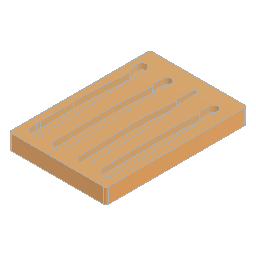
Tweezer-Carrier (Autodesk Fusion 360 design; units mm, degrees)
Autodesk Fusion 360 part; units mm, degrees
(part 1 of 2)
sketch "Sketch1" plane through (0, 0, 35.675) normal (0, 0, 1) x (-1, 0, 0)
  line L0 (-281.1, 293.942) -> (-205.1, 293.942)
  line L1 (-205.1, 293.942) -> (-205.1, 181.942)
  line L2 (-205.1, 181.942) -> (-281.1, 181.942)
  line L3 (-281.1, 181.942) -> (-281.1, 293.942)
  arc A0 (-205.1, 179.942) -> (-203.1, 181.942) centre (-205.1, 181.942) ccw
  line L4 (-203.1, 181.942) -> (-203.1, 293.942)
  arc A1 (-203.1, 293.942) -> (-205.1, 295.942) centre (-205.1, 293.942) ccw
  line L5 (-205.1, 295.942) -> (-281.1, 295.942)
  arc A2 (-281.1, 295.942) -> (-283.1, 293.942) centre (-281.1, 293.942) ccw
  line L6 (-283.1, 293.942) -> (-283.1, 181.942)
  arc A3 (-283.1, 181.942) -> (-281.1, 179.942) centre (-281.1, 181.942) ccw
  line L7 (-281.1, 179.942) -> (-205.1, 179.942)
  line L8 (-283.025, 293.942) -> (-283.025, 181.942)
  arc A4 (-283.025, 181.942) -> (-281.1, 180.017) centre (-281.1, 181.942) ccw
  line L9 (-281.1, 180.017) -> (-205.1, 180.017)
  arc A5 (-205.1, 180.017) -> (-203.175, 181.942) centre (-205.1, 181.942) ccw
  line L10 (-203.175, 181.942) -> (-203.175, 293.942)
  arc A6 (-203.175, 293.942) -> (-205.1, 295.867) centre (-205.1, 293.942) ccw
  line L11 (-205.1, 295.867) -> (-281.1, 295.867)
  arc A7 (-281.1, 295.867) -> (-283.025, 293.942) centre (-281.1, 293.942) ccw
  dimension "d162" = -0.075
extrude "Extrude1" add sketch "Sketch1" along normal blind 12.5 contours L0 L1 L2 L3 | L8 A4 L9 A5 L10 A6 L11 A7
sketch "Sketch2" plane through (0, 0, 48.175) normal (0, 0, 1) x (-1, 0, 0)
  arc A0 (-281.1, 295.867) -> (-283.025, 293.942) centre (-281.1, 293.942) ccw
  line L0 (-283.025, 293.942) -> (-283.025, 181.942)
  arc A1 (-283.025, 181.942) -> (-281.1, 180.017) centre (-281.1, 181.942) ccw
  line L1 (-281.1, 180.017) -> (-205.1, 180.017)
  arc A2 (-205.1, 180.017) -> (-203.175, 181.942) centre (-205.1, 181.942) ccw
  line L2 (-203.175, 181.942) -> (-203.175, 293.942)
  arc A3 (-203.175, 293.942) -> (-205.1, 295.867) centre (-205.1, 293.942) ccw
  line L3 (-205.1, 295.867) -> (-281.1, 295.867)
sketch "Sketch3" plane through (0, 0, 48.175) normal (0, 0, 1) x (-1, 0, 0)
  spline S0 degree 5 poles (-213.5459, 288.1293) (-213.4945, 288.1336) (-213.392, 288.1403) (-213.2392, 288.1448) (-213.0373, 288.1395) (-212.788, 288.1142) (-212.5418, 288.0705) (-212.2989, 288.0088) (-212.0595, 287.93) (-211.8239, 287.8356) (-211.5927, 287.7271) (-211.3661, 287.6064) (-211.1447, 287.475) (-210.929, 287.3345) (-210.7193, 287.1857) (-210.5161, 287.0295) (-210.3201, 286.8663) (-210.132, 286.6964) (-209.9529, 286.5201) (-209.7839, 286.3373) (-209.6265, 286.1478) (-209.4815, 285.9505) (-209.35, 285.7437) (-209.232, 285.5245) (-209.1273, 285.2896) (-209.0354, 285.0362) (-208.9554, 284.763) (-208.8863, 284.4709) (-208.8273, 284.1647) (-208.7775, 283.8515) (-208.7361, 283.5396) (-208.7023, 283.2363) (-208.6754, 282.9464) (-208.6547, 282.6709) (-208.6396, 282.4048) (-208.6295, 282.1406) (-208.6238, 281.8697) (-208.6217, 281.5848) (-208.6227, 281.2826) (-208.6261, 280.9654) (-208.6309, 280.64) (-208.6366, 280.3159) (-208.6424, 280.0035) (-208.6478, 279.713) (-208.6524, 279.4518) (-208.6559, 279.2244) (-208.6578, 279.0713) (-208.6586, 278.9729) (-208.6589, 278.9146) (-208.6591, 278.8873) knots 0 0 0 0 0 0 0.022222 0.044444 0.066667 0.088889 0.111111 0.133333 0.155556 0.177778 0.2 0.222222 0.244444 0.266667 0.288889 0.311111 0.333333 0.355556 0.377778 0.4 0.422222 0.444444 0.466667 0.488889 0.511111 0.533333 0.555556 0.577778 0.6 0.622222 0.644444 0.666667 0.688889 0.711111 0.733333 0.755556 0.777778 0.8 0.822222 0.844444 0.866667 0.888889 0.911111 0.933333 0.955556 0.977778 1 1 1 1 1 1
  spline S1 degree 5 poles (-208.6591, 278.8873) (-208.6588, 278.9046) (-208.6584, 278.9324) (-208.6579, 278.9537) (-208.6576, 278.9414) (-208.6579, 278.8572) (-208.6588, 278.7058) (-208.6603, 278.4928) (-208.6623, 278.2279) (-208.6648, 277.9222) (-208.6676, 277.5876) (-208.6708, 277.2352) (-208.6742, 276.8738) (-208.6778, 276.5093) (-208.6815, 276.1457) (-208.6854, 275.785) (-208.6886, 275.4997) (-208.691, 275.2877) (-208.6927, 275.1471) (-208.6935, 275.0771) knots 0 0 0 0 0 0 0.066667 0.133333 0.2 0.266667 0.333333 0.4 0.466667 0.533333 0.6 0.666667 0.733333 0.8 0.866667 0.933333 1 1 1 1 1 1
  spline S2 degree 5 poles (-208.6935, 275.0771) (-208.6936, 275.0186) (-208.6937, 274.9022) (-208.6943, 274.7292) (-208.6958, 274.5019) (-208.6987, 274.2215) (-208.7025, 273.9399) (-208.7066, 273.6464) (-208.7105, 273.3274) (-208.7137, 272.9745) (-208.7157, 272.59) (-208.717, 272.1953) (-208.7179, 271.82) (-208.7189, 271.4886) (-208.7196, 271.2097) (-208.719, 270.9594) (-208.7155, 270.6952) (-208.7074, 270.3748) (-208.6936, 269.977) (-208.6742, 269.5091) (-208.6496, 268.9944) (-208.6213, 268.4634) (-208.5907, 267.9451) (-208.56, 267.4558) (-208.5313, 266.9953) (-208.5068, 266.5529) (-208.488, 266.1123) (-208.4762, 265.6565) (-208.4715, 265.1727) (-208.4731, 264.6559) (-208.4796, 264.1063) (-208.489, 263.5285) (-208.4994, 262.9299) (-208.5091, 262.3195) (-208.5169, 261.7068) (-208.5219, 261.1003) (-208.5241, 260.5075) (-208.5234, 259.9343) (-208.5201, 259.3837) (-208.5145, 258.8563) (-208.507, 258.3486) (-208.4978, 257.8538) (-208.4873, 257.363) (-208.4756, 256.8669) (-208.463, 256.357) (-208.4498, 255.8268) (-208.4363, 255.2734) (-208.4229, 254.6965) (-208.4099, 254.0975) (-208.3977, 253.4794) (-208.3867, 252.8456) (-208.377, 252.1996) (-208.369, 251.5437) (-208.3628, 250.8798) (-208.3584, 250.2092) (-208.356, 249.5325) (-208.3555, 248.9866) (-208.3561, 248.5747) (-208.3569, 248.299) (-208.3573, 248.1609) knots 0 0 0 0 0 0 0.018182 0.036364 0.054545 0.072727 0.090909 0.109091 0.127273 0.145455 0.163636 0.181818 0.2 0.218182 0.236364 0.254545 0.272727 0.290909 0.309091 0.327273 0.345455 0.363636 0.381818 0.4 0.418182 0.436364 0.454545 0.472727 0.490909 0.509091 0.527273 0.545455 0.563636 0.581818 0.6 0.618182 0.636364 0.654545 0.672727 0.690909 0.709091 0.727273 0.745455 0.763636 0.781818 0.8 0.818182 0.836364 0.854545 0.872727 0.890909 0.909091 0.927273 0.945455 0.963636 0.981818 1 1 1 1 1 1
  spline S3 degree 5 poles (-208.3573, 248.1609) (-208.3602, 248.1208) (-208.3652, 248.0297) (-208.3703, 247.8598) (-208.3725, 247.5669) (-208.3678, 247.0952) (-208.3563, 246.533) (-208.3394, 245.9116) (-208.3191, 245.27) (-208.2977, 244.6446) (-208.2777, 244.0606) (-208.2614, 243.5208) (-208.251, 243.0003) (-208.2479, 242.4607) (-208.2534, 241.8621) (-208.2674, 241.1754) (-208.2891, 240.3959) (-208.3171, 239.54) (-208.3493, 238.6365) (-208.3839, 237.7205) (-208.4195, 236.8259) (-208.4555, 235.979) (-208.4923, 235.1896) (-208.532, 234.4502) (-208.5765, 233.7433) (-208.6279, 233.0464) (-208.6868, 232.339) (-208.7523, 231.6075) (-208.8209, 230.8526) (-208.8872, 230.0861) (-208.9456, 229.3261) (-208.991, 228.5915) (-209.0205, 227.8983) (-209.0343, 227.2537) (-209.0368, 226.6527) (-209.0348, 226.0821) (-209.0354, 225.5244) (-209.0449, 224.9611) (-209.0665, 224.3769) (-209.0999, 223.7617) (-209.143, 223.1093) (-209.1926, 222.4178) (-209.246, 221.6887) (-209.3016, 220.9271) (-209.3597, 220.1406) (-209.4214, 219.3378) (-209.488, 218.5274) (-209.5606, 217.7163) (-209.6393, 216.9087) (-209.7226, 216.1045) (-209.8074, 215.2995) (-209.8899, 214.4882) (-209.9662, 213.6659) (-210.033, 212.8304) (-210.0881, 211.9843) (-210.1314, 211.1375) (-210.1646, 210.3075) (-210.1912, 209.5148) (-210.2149, 208.7791) (-210.2394, 208.1151) (-210.2674, 207.5294) (-210.2999, 207.0151) (-210.3363, 206.5533) (-210.3747, 206.1204) (-210.4135, 205.6932) (-210.4514, 205.2566) (-210.4804, 204.8939) (-210.5014, 204.6132) (-210.515, 204.4223) (-210.5217, 204.3258) knots 0 0 0 0 0 0 0.01538462 0.03076923 0.04615385 0.06153846 0.07692308 0.09230769 0.10769231 0.12307692 0.13846154 0.15384615 0.16923077 0.18461538 0.2 0.21538462 0.23076923 0.24615385 0.26153846 0.27692308 0.29230769 0.30769231 0.32307692 0.33846154 0.35384615 0.36923077 0.38461538 0.4 0.41538462 0.43076923 0.44615385 0.46153846 0.47692308 0.49230769 0.50769231 0.52307692 0.53846154 0.55384615 0.56923077 0.58461538 0.6 0.61538462 0.63076923 0.64615385 0.66153846 0.67692308 0.69230769 0.70769231 0.72307692 0.73846154 0.75384615 0.76923077 0.78461538 0.8 0.81538462 0.83076923 0.84615385 0.86153846 0.87692308 0.89230769 0.90769231 0.92307692 0.93846154 0.95384615 0.96923077 0.98461538 1 1 1 1 1 1
  spline S4 degree 5 poles (-210.5217, 204.3258) (-210.5153, 204.3258) (-210.5025, 204.3257) (-210.4832, 204.3256) (-210.4576, 204.3254) (-210.4255, 204.3252) (-210.3998, 204.325) (-210.3805, 204.3248) (-210.3677, 204.3248) (-210.3613, 204.3247) knots 0 0 0 0 0 0 0.2 0.4 0.6 0.8 1 1 1 1 1 1
  spline S5 degree 5 poles (-233.3855, 288.3655) (-233.3109, 288.3868) (-233.1597, 288.4223) (-232.9269, 288.4544) (-232.6048, 288.4548) (-232.1838, 288.3864) (-231.7481, 288.2539) (-231.3053, 288.0677) (-230.8655, 287.8391) (-230.4388, 287.5764) (-230.0337, 287.2794) (-229.6557, 286.937) (-229.3093, 286.5403) (-229, 286.0916) (-228.7363, 285.6179) (-228.53, 285.1713) (-228.3889, 284.7958) (-228.3129, 284.5049) (-228.2864, 284.2462) (-228.2853, 283.9325) (-228.2909, 283.5017) (-228.2958, 282.9438) (-228.299, 282.279) (-228.3035, 281.5446) (-228.3126, 280.779) (-228.3271, 280.007) (-228.3456, 279.2426) (-228.3656, 278.4911) (-228.3842, 277.7515) (-228.3986, 277.0193) (-228.407, 276.2886) (-228.4091, 275.554) (-228.4051, 274.811) (-228.3963, 274.0567) (-228.384, 273.2907) (-228.3695, 272.5152) (-228.354, 271.7363) (-228.3381, 270.962) (-228.3224, 270.2004) (-228.307, 269.4576) (-228.2923, 268.7359) (-228.2782, 268.0318) (-228.2647, 267.3348) (-228.2518, 266.6317) (-228.2394, 265.9094) (-228.2275, 265.1587) (-228.2159, 264.3769) (-228.2046, 263.5719) (-228.1935, 262.7581) (-228.1826, 261.9529) (-228.1719, 261.1721) (-228.1613, 260.4259) (-228.1509, 259.715) (-228.1408, 259.0267) (-228.1311, 258.341) (-228.1219, 257.6352) (-228.1133, 256.8893) (-228.1054, 256.091) (-228.0982, 255.2416) (-228.0917, 254.3536) (-228.0858, 253.4464) (-228.0805, 252.542) (-228.0759, 251.6609) (-228.0719, 250.8182) (-228.0686, 250.019) (-228.0661, 249.2565) (-228.0646, 248.5169) (-228.0641, 247.7823) (-228.0646, 247.0346) (-228.066, 246.2591) (-228.0678, 245.4479) (-228.0694, 244.6008) (-228.0704, 243.723) (-228.07, 242.8238) (-228.0679, 241.9156) (-228.0637, 241.0121) (-228.0575, 240.1271) (-228.0496, 239.2735) (-228.0406, 238.461) (-228.0316, 237.6958) (-228.0235, 236.9786) (-228.0179, 236.3035) (-228.0161, 235.6561) (-228.0198, 235.0147) (-228.0301, 234.356) (-228.0478, 233.6596) (-228.0726, 232.913) (-228.1029, 232.1172) (-228.136, 231.2881) (-228.1687, 230.4489) (-228.1982, 229.6258) (-228.2224, 228.8413) (-228.2409, 228.1096) (-228.256, 227.4294) (-228.2719, 226.7838) (-228.2938, 226.1483) (-228.3263, 225.4969) (-228.3722, 224.8084) (-228.4309, 224.074) (-228.4985, 223.2987) (-228.5694, 222.4953) (-228.6375, 221.6812) (-228.6978, 220.8734) (-228.7474, 220.085) (-228.7877, 219.3194) (-228.823, 218.5722) (-228.8592, 217.8345) (-228.902, 217.0958) (-228.9558, 216.3473) (-229.0216, 215.5849) (-229.0961, 214.8119) (-229.1733, 214.0367) (-229.246, 213.2705) (-229.3073, 212.5252) (-229.3522, 211.8116) (-229.3792, 211.1364) (-229.3909, 210.5019) (-229.3919, 209.9061) (-229.3881, 209.3436) (-229.3851, 208.8058) (-229.387, 208.2812) (-229.3961, 207.7568) (-229.4141, 207.2199) (-229.4415, 206.6592) (-229.4788, 206.0671) (-229.5264, 205.439) (-229.5728, 204.906) (-229.6122, 204.4886) (-229.6406, 204.2026) (-229.6553, 204.0577) knots 0 0 0 0 0 0 0.008 0.016 0.024 0.032 0.04 0.048 0.056 0.064 0.072 0.08 0.088 0.096 0.104 0.112 0.12 0.128 0.136 0.144 0.152 0.16 0.168 0.176 0.184 0.192 0.2 0.208 0.216 0.224 0.232 0.24 0.248 0.256 0.264 0.272 0.28 0.288 0.296 0.304 0.312 0.32 0.328 0.336 0.344 0.352 0.36 0.368 0.376 0.384 0.392 0.4 0.408 0.416 0.424 0.432 0.44 0.448 0.456 0.464 0.472 0.48 0.488 0.496 0.504 0.512 0.52 0.528 0.536 0.544 0.552 0.56 0.568 0.576 0.584 0.592 0.6 0.608 0.616 0.624 0.632 0.64 0.648 0.656 0.664 0.672 0.68 0.688 0.696 0.704 0.712 0.72 0.728 0.736 0.744 0.752 0.76 0.768 0.776 0.784 0.792 0.8 0.808 0.816 0.824 0.832 0.84 0.848 0.856 0.864 0.872 0.88 0.888 0.896 0.904 0.912 0.92 0.928 0.936 0.944 0.952 0.96 0.968 0.976 0.984 0.992 1 1 1 1 1 1
  spline S6 degree 5 poles (-229.6553, 204.0577) (-229.6247, 204.0624) (-229.563, 204.0703) (-229.4689, 204.0774) (-229.3402, 204.0777) (-229.1753, 204.0615) (-229.0101, 204.0253) (-228.8525, 203.9625) (-228.7115, 203.8646) (-228.595, 203.723) (-228.5063, 203.5311) (-228.4442, 203.285) (-228.4052, 202.9837) (-228.3843, 202.6298) (-228.3765, 202.2298) (-228.3776, 201.7942) (-228.3842, 201.3354) (-228.3935, 200.8667) (-228.4033, 200.4009) (-228.412, 199.9484) (-228.4189, 199.5165) (-228.4236, 199.1069) (-228.4265, 198.7162) (-228.4282, 198.3371) (-228.4295, 197.9607) (-228.4311, 197.5782) (-228.4335, 197.1823) (-228.4368, 196.7698) (-228.4401, 196.3426) (-228.4429, 195.9069) (-228.4444, 195.4714) (-228.4451, 195.0458) (-228.4467, 194.6392) (-228.4527, 194.2582) (-228.4692, 193.9059) (-228.505, 193.58) (-228.5691, 193.2757) (-228.6686, 192.9873) (-228.8065, 192.7103) (-228.9798, 192.4437) (-229.1763, 192.1917) (-229.3792, 191.9626) (-229.5726, 191.7655) (-229.7468, 191.6078) (-229.9033, 191.493) (-230.0608, 191.4178) (-230.2434, 191.3746) (-230.4717, 191.3535) (-230.7492, 191.3447) (-231.0615, 191.3404) (-231.3856, 191.3348) (-231.6972, 191.3251) (-231.9778, 191.3124) (-232.2241, 191.3026) (-232.4476, 191.3053) (-232.6653, 191.3308) (-232.8945, 191.3882) (-233.144, 191.482) (-233.4112, 191.6116) (-233.6874, 191.7735) (-233.9599, 191.9626) (-234.2162, 192.1743) (-234.4471, 192.4064) (-234.6486, 192.6598) (-234.8203, 192.9367) (-234.9643, 193.24) (-235.0837, 193.572) (-235.1819, 193.9335) (-235.2611, 194.3223) (-235.3225, 194.7341) (-235.367, 195.1637) (-235.3953, 195.6055) (-235.4085, 196.0549) (-235.4082, 196.5085) (-235.3972, 196.9655) (-235.3794, 197.4284) (-235.3597, 197.9013) (-235.343, 198.3892) (-235.3344, 198.8963) (-235.3378, 199.4251) (-235.3563, 199.9749) (-235.3911, 200.5409) (-235.4414, 201.1126) (-235.5035, 201.673) (-235.5717, 202.2018) (-235.6389, 202.6781) (-235.6969, 203.0834) (-235.7369, 203.405) (-235.7502, 203.6386) (-235.7289, 203.7915) (-235.6658, 203.8856) (-235.5581, 203.9484) (-235.4111, 204.001) (-235.2393, 204.0517) (-235.0601, 204.1017) (-234.8882, 204.1493) (-234.7623, 204.1849) (-234.6755, 204.21) (-234.621, 204.2261) (-234.5946, 204.234) knots 0 0 0 0 0 0 0.01052632 0.02105263 0.03157895 0.04210526 0.05263158 0.06315789 0.07368421 0.08421053 0.09473684 0.10526316 0.11578947 0.12631579 0.13684211 0.14736842 0.15789474 0.16842105 0.17894737 0.18947368 0.2 0.21052632 0.22105263 0.23157895 0.24210526 0.25263158 0.26315789 0.27368421 0.28421053 0.29473684 0.30526316 0.31578947 0.32631579 0.33684211 0.34736842 0.35789474 0.36842105 0.37894737 0.38947368 0.4 0.41052632 0.42105263 0.43157895 0.44210526 0.45263158 0.46315789 0.47368421 0.48421053 0.49473684 0.50526316 0.51578947 0.52631579 0.53684211 0.54736842 0.55789474 0.56842105 0.57894737 0.58947368 0.6 0.61052632 0.62105263 0.63157895 0.64210526 0.65263158 0.66315789 0.67368421 0.68421053 0.69473684 0.70526316 0.71578947 0.72631579 0.73684211 0.74736842 0.75789474 0.76842105 0.77894737 0.78947368 0.8 0.81052632 0.82105263 0.83157895 0.84210526 0.85263158 0.86315789 0.87368421 0.88421053 0.89473684 0.90526316 0.91578947 0.92631579 0.93684211 0.94736842 0.95789474 0.96842105 0.97894737 0.98947368 1 1 1 1 1 1
  spline S7 degree 5 poles (-234.5946, 204.234) (-234.611, 204.3872) (-234.6431, 204.6936) (-234.6891, 205.1525) (-234.7462, 205.7631) (-234.8105, 206.525) (-234.8685, 207.2874) (-234.9212, 208.0541) (-234.9708, 208.8316) (-235.0201, 209.6287) (-235.0719, 210.4544) (-235.129, 211.3153) (-235.193, 212.2139) (-235.2642, 213.146) (-235.3411, 214.1003) (-235.4214, 215.0623) (-235.5025, 216.0167) (-235.5817, 216.9508) (-235.6574, 217.8567) (-235.7291, 218.7354) (-235.7979, 219.5944) (-235.8652, 220.445) (-235.933, 221.2984) (-236.0028, 222.1639) (-236.0759, 223.0445) (-236.1525, 223.9371) (-236.2325, 224.8356) (-236.3151, 225.733) (-236.3993, 226.6238) (-236.4834, 227.5063) (-236.566, 228.3848) (-236.6455, 229.2663) (-236.7204, 230.1594) (-236.79, 231.0718) (-236.8538, 232.008) (-236.9124, 232.9676) (-236.9672, 233.946) (-237.0195, 234.9362) (-237.0711, 235.9308) (-237.1234, 236.9227) (-237.1772, 237.9079) (-237.2328, 238.8861) (-237.2895, 239.8601) (-237.3464, 240.8345) (-237.4022, 241.815) (-237.4554, 242.8069) (-237.5043, 243.8142) (-237.5476, 244.8386) (-237.5838, 245.8798) (-237.6123, 246.9357) (-237.6326, 248.0024) (-237.645, 249.0741) (-237.6506, 250.144) (-237.6515, 251.2035) (-237.6503, 252.244) (-237.6499, 253.2578) (-237.6529, 254.2393) (-237.6618, 255.1862) (-237.6779, 256.1006) (-237.7014, 256.9906) (-237.7315, 257.8675) (-237.7666, 258.7431) (-237.8049, 259.6271) (-237.8443, 260.524) (-237.883, 261.4301) (-237.9195, 262.334) (-237.9529, 263.2222) (-237.9823, 264.0827) (-238.0071, 264.9091) (-238.0273, 265.7056) (-238.043, 266.4885) (-238.0547, 267.2803) (-238.0632, 268.1032) (-238.0699, 268.9747) (-238.0766, 269.9005) (-238.0854, 270.8726) (-238.0983, 271.8754) (-238.1168, 272.8894) (-238.1416, 273.8964) (-238.1718, 274.8836) (-238.2048, 275.849) (-238.2366, 276.8006) (-238.2628, 277.75) (-238.2798, 278.7077) (-238.2863, 279.6776) (-238.2836, 280.652) (-238.2775, 281.6054) (-238.2741, 282.5022) (-238.2746, 283.3085) (-238.2692, 284.003) (-238.2338, 284.5855) (-238.1206, 285.0929) (-237.8801, 285.5783) (-237.4904, 286.0822) (-236.9907, 286.5999) (-236.4884, 287.0711) (-236.0878, 287.4297) (-235.8432, 287.6352) (-235.6805, 287.7263) (-235.4402, 287.7959) (-235.0162, 287.9058) (-234.4897, 288.0497) (-233.9816, 288.1936) (-233.5926, 288.3056) (-233.3855, 288.3655) knots 0 0 0 0 0 0 0.01 0.02 0.03 0.04 0.05 0.06 0.07 0.08 0.09 0.1 0.11 0.12 0.13 0.14 0.15 0.16 0.17 0.18 0.19 0.2 0.21 0.22 0.23 0.24 0.25 0.26 0.27 0.28 0.29 0.3 0.31 0.32 0.33 0.34 0.35 0.36 0.37 0.38 0.39 0.4 0.41 0.42 0.43 0.44 0.45 0.46 0.47 0.48 0.49 0.5 0.51 0.52 0.53 0.54 0.55 0.56 0.57 0.58 0.59 0.6 0.61 0.62 0.63 0.64 0.65 0.66 0.67 0.68 0.69 0.7 0.71 0.72 0.73 0.74 0.75 0.76 0.77 0.78 0.79 0.8 0.81 0.82 0.83 0.84 0.85 0.86 0.87 0.88 0.89 0.9 0.91 0.92 0.93 0.94 0.95 0.96 0.97 0.98 0.99 1 1 1 1 1 1
  spline S8 degree 5 poles (-251.1217, 189.6278) (-251.0472, 189.6102) (-250.9024, 189.5836) (-250.6981, 189.57) (-250.4517, 189.6043) (-250.1865, 189.7344) (-249.9635, 189.951) (-249.7806, 190.2515) (-249.6345, 190.6314) (-249.5209, 191.0843) (-249.435, 191.6012) (-249.3718, 192.1712) (-249.3265, 192.7806) (-249.2947, 193.4137) (-249.2725, 194.0547) (-249.2564, 194.6891) (-249.2436, 195.3058) (-249.2316, 195.8979) (-249.2186, 196.4656) (-249.2036, 197.0168) (-249.1858, 197.5643) (-249.1649, 198.1228) (-249.141, 198.7054) (-249.114, 199.3204) (-249.0841, 199.9682) (-249.051, 200.6379) (-249.015, 201.3107) (-248.9769, 201.9639) (-248.9389, 202.5743) (-248.9049, 203.1218) (-248.8809, 203.5929) (-248.8758, 203.9853) (-248.9006, 204.307) (-248.9666, 204.5713) (-249.0837, 204.7924) (-249.2583, 204.9804) (-249.4464, 205.1083) (-249.6151, 205.1923) (-249.7397, 205.243) (-249.8051, 205.267) knots 0 0 0 0 0 0 0.028571 0.057143 0.085714 0.114286 0.142857 0.171429 0.2 0.228571 0.257143 0.285714 0.314286 0.342857 0.371429 0.4 0.428571 0.457143 0.485714 0.514286 0.542857 0.571429 0.6 0.628571 0.657143 0.685714 0.714286 0.742857 0.771429 0.8 0.828571 0.857143 0.885714 0.914286 0.942857 0.971429 1 1 1 1 1 1
  spline S9 degree 5 poles (-251.1217, 189.6278) (-251.1499, 189.624) (-251.2071, 189.6195) (-251.295, 189.6225) (-251.4163, 189.6458) (-251.5742, 189.707) (-251.7369, 189.7994) (-251.9013, 189.9211) (-252.0626, 190.0696) (-252.2157, 190.2423) (-252.3559, 190.4377) (-252.4799, 190.656) (-252.5867, 190.8998) (-252.6764, 191.1726) (-252.7508, 191.4781) (-252.8118, 191.8188) (-252.862, 192.1952) (-252.9036, 192.6042) (-252.9386, 193.0404) (-252.9687, 193.4965) (-252.9955, 193.9646) (-253.0203, 194.4369) (-253.0442, 194.9067) (-253.0682, 195.3696) (-253.0929, 195.8239) (-253.119, 196.2718) (-253.1468, 196.7179) (-253.1765, 197.1684) (-253.2083, 197.6294) (-253.2421, 198.1065) (-253.278, 198.6031) (-253.3156, 199.1196) (-253.3548, 199.6524) (-253.3952, 200.1922) (-253.4367, 200.7266) (-253.4791, 201.2414) (-253.5224, 201.722) (-253.5672, 202.1554) (-253.614, 202.5316) (-253.6642, 202.8456) (-253.7194, 203.0986) (-253.782, 203.3) (-253.8534, 203.4641) (-253.9325, 203.6077) (-254.0145, 203.7468) (-254.0887, 203.8942) (-254.1425, 204.0571) (-254.165, 204.236) (-254.1513, 204.4219) (-254.105, 204.5968) (-254.033, 204.7416) (-253.9429, 204.8421) (-253.8384, 204.8979) (-253.7194, 204.9195) (-253.5842, 204.921) (-253.4313, 204.9125) (-253.2944, 204.9014) (-253.1834, 204.8915) (-253.1056, 204.8842) (-253.0659, 204.8803) knots 0 0 0 0 0 0 0.018182 0.036364 0.054545 0.072727 0.090909 0.109091 0.127273 0.145455 0.163636 0.181818 0.2 0.218182 0.236364 0.254545 0.272727 0.290909 0.309091 0.327273 0.345455 0.363636 0.381818 0.4 0.418182 0.436364 0.454545 0.472727 0.490909 0.509091 0.527273 0.545455 0.563636 0.581818 0.6 0.618182 0.636364 0.654545 0.672727 0.690909 0.709091 0.727273 0.745455 0.763636 0.781818 0.8 0.818182 0.836364 0.854545 0.872727 0.890909 0.909091 0.927273 0.945455 0.963636 0.981818 1 1 1 1 1 1
  spline S10 degree 5 poles (-254.3567, 288.4328) (-254.2692, 288.4344) (-254.0999, 288.435) (-253.8631, 288.4277) (-253.5819, 288.4019) (-253.2812, 288.3428) (-253.0109, 288.2568) (-252.7308, 288.1439) (-252.4023, 288.0034) (-252.0152, 287.8327) (-251.6003, 287.6276) (-251.2011, 287.3857) (-250.8556, 287.1087) (-250.5679, 286.8064) (-250.3163, 286.494) (-250.0745, 286.1853) (-249.8331, 285.8875) (-249.6104, 285.597) (-249.4318, 285.3025) (-249.3133, 284.987) (-249.2479, 284.6307) (-249.2178, 284.2158) (-249.2038, 283.7313) (-249.1952, 283.1778) (-249.1867, 282.5639) (-249.1773, 281.9027) (-249.1679, 281.2092) (-249.1592, 280.4964) (-249.1508, 279.7731) (-249.1416, 279.0453) (-249.13, 278.3165) (-249.1148, 277.588) (-249.095, 276.8599) (-249.0707, 276.1315) (-249.0427, 275.4016) (-249.0128, 274.6687) (-248.9827, 273.9308) (-248.954, 273.186) (-248.9281, 272.432) (-248.9055, 271.6667) (-248.8861, 270.8883) (-248.8691, 270.0962) (-248.8536, 269.2911) (-248.8387, 268.4757) (-248.8235, 267.6557) (-248.8076, 266.8397) (-248.7911, 266.0396) (-248.7743, 265.2672) (-248.7576, 264.5324) (-248.7415, 263.841) (-248.7264, 263.1922) (-248.7124, 262.5757) (-248.6991, 261.9726) (-248.6859, 261.3621) (-248.6721, 260.727) (-248.6568, 260.0595) (-248.639, 259.368) (-248.6176, 258.6784) (-248.5921, 258.0229) (-248.5623, 257.4313) (-248.5288, 256.9218) (-248.4934, 256.4907) (-248.4588, 256.1082) (-248.428, 255.7346) (-248.4038, 255.333) (-248.3877, 254.8846) (-248.3801, 254.3856) (-248.3804, 253.8412) (-248.3866, 253.2609) (-248.396, 252.6524) (-248.405, 252.0222) (-248.4103, 251.375) (-248.4092, 250.7137) (-248.4001, 250.0399) (-248.3831, 249.3533) (-248.3598, 248.6526) (-248.3326, 247.9357) (-248.3042, 247.2005) (-248.2771, 246.4453) (-248.2529, 245.6693) (-248.2322, 244.873) (-248.2147, 244.0583) (-248.1998, 243.2279) (-248.1863, 242.386) (-248.1734, 241.5373) (-248.1602, 240.6875) (-248.1467, 239.8433) (-248.1333, 239.0113) (-248.1208, 238.1977) (-248.1102, 237.4074) (-248.1024, 236.6433) (-248.0985, 235.9055) (-248.0991, 235.1903) (-248.1046, 234.4905) (-248.115, 233.7969) (-248.1303, 233.0997) (-248.1503, 232.3903) (-248.1746, 231.6624) (-248.2029, 230.9141) (-248.2349, 230.1474) (-248.2706, 229.3665) (-248.3095, 228.5769) (-248.3516, 227.7842) (-248.3968, 226.9926) (-248.4448, 226.2039) (-248.4957, 225.417) (-248.5493, 224.6295) (-248.6053, 223.8383) (-248.6633, 223.0405) (-248.7227, 222.2346) (-248.7826, 221.4216) (-248.8418, 220.6052) (-248.8991, 219.7906) (-248.9532, 218.9837) (-249.0032, 218.1893) (-249.0486, 217.4108) (-249.0892, 216.6484) (-249.1261, 215.8979) (-249.1604, 215.1523) (-249.194, 214.4033) (-249.2286, 213.6431) (-249.2657, 212.8663) (-249.3063, 212.0713) (-249.351, 211.2625) (-249.3992, 210.4493) (-249.4502, 209.6443) (-249.503, 208.8616) (-249.5565, 208.1154) (-249.6095, 207.4182) (-249.6612, 206.779) (-249.7113, 206.2032) (-249.7498, 205.7953) (-249.7778, 205.5195) (-249.7961, 205.349) (-249.8051, 205.267) knots 0 0 0 0 0 0 0.00769231 0.01538462 0.02307692 0.03076923 0.03846154 0.04615385 0.05384615 0.06153846 0.06923077 0.07692308 0.08461538 0.09230769 0.1 0.10769231 0.11538462 0.12307692 0.13076923 0.13846154 0.14615385 0.15384615 0.16153846 0.16923077 0.17692308 0.18461538 0.19230769 0.2 0.20769231 0.21538462 0.22307692 0.23076923 0.23846154 0.24615385 0.25384615 0.26153846 0.26923077 0.27692308 0.28461538 0.29230769 0.3 0.30769231 0.31538462 0.32307692 0.33076923 0.33846154 0.34615385 0.35384615 0.36153846 0.36923077 0.37692308 0.38461538 0.39230769 0.4 0.40769231 0.41538462 0.42307692 0.43076923 0.43846154 0.44615385 0.45384615 0.46153846 0.46923077 0.47692308 0.48461538 0.49230769 0.5 0.50769231 0.51538462 0.52307692 0.53076923 0.53846154 0.54615385 0.55384615 0.56153846 0.56923077 0.57692308 0.58461538 0.59230769 0.6 0.60769231 0.61538462 0.62307692 0.63076923 0.63846154 0.64615385 0.65384615 0.66153846 0.66923077 0.67692308 0.68461538 0.69230769 0.7 0.70769231 0.71538462 0.72307692 0.73076923 0.73846154 0.74615385 0.75384615 0.76153846 0.76923077 0.77692308 0.78461538 0.79230769 0.8 0.80769231 0.81538462 0.82307692 0.83076923 0.83846154 0.84615385 0.85384615 0.86153846 0.86923077 0.87692308 0.88461538 0.89230769 0.9 0.90769231 0.91538462 0.92307692 0.93076923 0.93846154 0.94615385 0.95384615 0.96153846 0.96923077 0.97692308 0.98461538 0.99230769 1 1 1 1 1 1
  spline S11 degree 5 poles (-254.3567, 288.4328) (-254.4631, 288.4521) (-254.6744, 288.4769) (-254.9863, 288.4731) (-255.3923, 288.3858) (-255.8836, 288.1455) (-256.3585, 287.7914) (-256.8175, 287.3595) (-257.2594, 286.8952) (-257.6798, 286.4374) (-258.0685, 286.0052) (-258.4081, 285.5834) (-258.6806, 285.1414) (-258.8736, 284.6485) (-258.9884, 284.0953) (-259.0387, 283.4922) (-259.0431, 282.8563) (-259.0202, 282.2018) (-258.9823, 281.5295) (-258.9378, 280.8333) (-258.8912, 280.1052) (-258.845, 279.3403) (-258.8008, 278.5431) (-258.7592, 277.7238) (-258.7203, 276.8948) (-258.6838, 276.0664) (-258.6495, 275.243) (-258.617, 274.4197) (-258.586, 273.5857) (-258.5562, 272.7284) (-258.5273, 271.8367) (-258.4986, 270.905) (-258.4696, 269.9362) (-258.4394, 268.94) (-258.4072, 267.9291) (-258.3727, 266.917) (-258.3353, 265.9147) (-258.2953, 264.9282) (-258.2532, 263.9562) (-258.2099, 262.9923) (-258.1663, 262.0276) (-258.1232, 261.0529) (-258.0812, 260.0612) (-258.0401, 259.0498) (-257.9995, 258.0219) (-257.9584, 256.9845) (-257.9159, 255.9467) (-257.8711, 254.9181) (-257.8237, 253.9075) (-257.774, 252.9208) (-257.7233, 251.9603) (-257.6732, 251.0251) (-257.6253, 250.1119) (-257.5814, 249.2159) (-257.5424, 248.3309) (-257.5086, 247.4502) (-257.4794, 246.5673) (-257.4537, 245.6766) (-257.43, 244.774) (-257.4067, 243.8578) (-257.3825, 242.9293) (-257.356, 241.993) (-257.3264, 241.0557) (-257.2928, 240.125) (-257.2545, 239.2086) (-257.2109, 238.313) (-257.1612, 237.4426) (-257.1048, 236.5992) (-257.0412, 235.7818) (-256.9698, 234.9862) (-256.8903, 234.2049) (-256.8026, 233.4266) (-256.7069, 232.638) (-256.6035, 231.8264) (-256.4935, 230.9824) (-256.3782, 230.1018) (-256.2596, 229.1887) (-256.14, 228.253) (-256.0215, 227.3069) (-255.9059, 226.3626) (-255.7941, 225.429) (-255.6856, 224.5091) (-255.5788, 223.5984) (-255.4713, 222.6885) (-255.3607, 221.7693) (-255.2445, 220.8318) (-255.1213, 219.8707) (-254.991, 218.8868) (-254.8544, 217.8861) (-254.7132, 216.8776) (-254.5695, 215.8717) (-254.4255, 214.8779) (-254.2831, 213.9034) (-254.1435, 212.951) (-254.0076, 212.0199) (-253.8757, 211.1067) (-253.7479, 210.2069) (-253.6243, 209.3153) (-253.5046, 208.428) (-253.3889, 207.5421) (-253.277, 206.656) (-253.1906, 205.9464) (-253.1276, 205.4136) (-253.0863, 205.0581) (-253.0659, 204.8803) knots 0 0 0 0 0 0 0.01 0.02 0.03 0.04 0.05 0.06 0.07 0.08 0.09 0.1 0.11 0.12 0.13 0.14 0.15 0.16 0.17 0.18 0.19 0.2 0.21 0.22 0.23 0.24 0.25 0.26 0.27 0.28 0.29 0.3 0.31 0.32 0.33 0.34 0.35 0.36 0.37 0.38 0.39 0.4 0.41 0.42 0.43 0.44 0.45 0.46 0.47 0.48 0.49 0.5 0.51 0.52 0.53 0.54 0.55 0.56 0.57 0.58 0.59 0.6 0.61 0.62 0.63 0.64 0.65 0.66 0.67 0.68 0.69 0.7 0.71 0.72 0.73 0.74 0.75 0.76 0.77 0.78 0.79 0.8 0.81 0.82 0.83 0.84 0.85 0.86 0.87 0.88 0.89 0.9 0.91 0.92 0.93 0.94 0.95 0.96 0.97 0.98 0.99 1 1 1 1 1 1
  spline S12 degree 5 poles (-272.7173, 288.4864) (-272.632, 288.5001) (-272.46, 288.5217) (-272.1981, 288.5368) (-271.8414, 288.5221) (-271.3844, 288.4468) (-270.9205, 288.3177) (-270.4587, 288.1409) (-270.0122, 287.9255) (-269.5941, 287.6792) (-269.2145, 287.4068) (-268.8764, 287.1055) (-268.5772, 286.7677) (-268.3121, 286.3852) (-268.0771, 285.9539) (-267.8719, 285.4771) (-267.6981, 284.9625) (-267.557, 284.4199) (-267.449, 283.8585) (-267.3712, 283.2847) (-267.3187, 282.7026) (-267.2859, 282.1141) (-267.2672, 281.5201) (-267.2578, 280.9201) (-267.2546, 280.3131) (-267.2552, 279.6981) (-267.2579, 279.0741) (-267.2614, 278.4406) (-267.2644, 277.7981) (-267.2659, 277.1479) (-267.265, 276.4918) (-267.2612, 275.8315) (-267.2541, 275.1689) (-267.244, 274.5056) (-267.2315, 273.8426) (-267.2173, 273.1803) (-267.2022, 272.5187) (-267.187, 271.8569) (-267.1722, 271.1931) (-267.1582, 270.5251) (-267.1453, 269.8513) (-267.1335, 269.1706) (-267.1225, 268.4839) (-267.112, 267.7939) (-267.1016, 267.1054) (-267.0906, 266.4231) (-267.0786, 265.7513) (-267.0654, 265.0924) (-267.0509, 264.4458) (-267.0356, 263.8079) (-267.0201, 263.1741) (-267.0053, 262.5394) (-266.9924, 261.9003) (-266.9829, 261.256) (-266.9783, 260.6084) (-266.9797, 259.96) (-266.9874, 259.3133) (-267.0006, 258.669) (-267.0169, 258.0252) (-267.0328, 257.377) (-267.0445, 256.7196) (-267.0489, 256.0487) (-267.0444, 255.3626) (-267.0316, 254.6641) (-267.0134, 253.9593) (-266.9935, 253.2561) (-266.9756, 252.5618) (-266.9625, 251.8818) (-266.9551, 251.2173) (-266.9516, 250.5648) (-266.9493, 249.9177) (-266.9452, 249.2679) (-266.937, 248.6073) (-266.9241, 247.9291) (-266.9082, 247.2294) (-266.8921, 246.5071) (-266.8789, 245.7652) (-266.8715, 245.0106) (-266.8715, 244.2552) (-266.8782, 243.5163) (-266.8895, 242.8129) (-266.9029, 242.1609) (-266.9156, 241.5689) (-266.926, 241.0339) (-266.9339, 240.5355) (-266.941, 240.0414) (-266.9494, 239.5174) (-266.9612, 238.9348) (-266.9777, 238.2816) (-266.9992, 237.5612) (-267.0256, 236.7877) (-267.0561, 235.981) (-267.0897, 235.1628) (-267.1251, 234.3519) (-267.1612, 233.56) (-267.1971, 232.7932) (-267.2318, 232.0528) (-267.2644, 231.3361) (-267.2943, 230.6376) (-267.3211, 229.9495) (-267.3444, 229.2631) (-267.3641, 228.5694) (-267.3805, 227.8602) (-267.3939, 227.1286) (-267.405, 226.3705) (-267.4148, 225.5849) (-267.4244, 224.7737) (-267.4353, 223.9407) (-267.4485, 223.0913) (-267.4652, 222.2311) (-267.4863, 221.3663) (-267.5122, 220.5018) (-267.5432, 219.642) (-267.5791, 218.7898) (-267.6196, 217.9472) (-267.6642, 217.1148) (-267.7122, 216.2918) (-267.7629, 215.4757) (-267.8155, 214.6629) (-267.8693, 213.849) (-267.9234, 213.0304) (-267.9772, 212.2051) (-268.0301, 211.3734) (-268.0816, 210.5391) (-268.1316, 209.7103) (-268.1797, 208.8975) (-268.2261, 208.1133) (-268.2708, 207.3698) (-268.3137, 206.6784) (-268.3549, 206.0479) (-268.3946, 205.4834) (-268.425, 205.0866) (-268.4471, 204.8203) (-268.4616, 204.6566) (-268.4687, 204.5782) knots 0 0 0 0 0 0 0.00769231 0.01538462 0.02307692 0.03076923 0.03846154 0.04615385 0.05384615 0.06153846 0.06923077 0.07692308 0.08461538 0.09230769 0.1 0.10769231 0.11538462 0.12307692 0.13076923 0.13846154 0.14615385 0.15384615 0.16153846 0.16923077 0.17692308 0.18461538 0.19230769 0.2 0.20769231 0.21538462 0.22307692 0.23076923 0.23846154 0.24615385 0.25384615 0.26153846 0.26923077 0.27692308 0.28461538 0.29230769 0.3 0.30769231 0.31538462 0.32307692 0.33076923 0.33846154 0.34615385 0.35384615 0.36153846 0.36923077 0.37692308 0.38461538 0.39230769 0.4 0.40769231 0.41538462 0.42307692 0.43076923 0.43846154 0.44615385 0.45384615 0.46153846 0.46923077 0.47692308 0.48461538 0.49230769 0.5 0.50769231 0.51538462 0.52307692 0.53076923 0.53846154 0.54615385 0.55384615 0.56153846 0.56923077 0.57692308 0.58461538 0.59230769 0.6 0.60769231 0.61538462 0.62307692 0.63076923 0.63846154 0.64615385 0.65384615 0.66153846 0.66923077 0.67692308 0.68461538 0.69230769 0.7 0.70769231 0.71538462 0.72307692 0.73076923 0.73846154 0.74615385 0.75384615 0.76153846 0.76923077 0.77692308 0.78461538 0.79230769 0.8 0.80769231 0.81538462 0.82307692 0.83076923 0.83846154 0.84615385 0.85384615 0.86153846 0.86923077 0.87692308 0.88461538 0.89230769 0.9 0.90769231 0.91538462 0.92307692 0.93076923 0.93846154 0.94615385 0.95384615 0.96153846 0.96923077 0.97692308 0.98461538 0.99230769 1 1 1 1 1 1
  spline S13 degree 5 poles (-272.7173, 288.4864) (-272.8609, 288.4558) (-273.1449, 288.3876) (-273.5613, 288.2648) (-274.0971, 288.06) (-274.7313, 287.7342) (-275.3194, 287.3346) (-275.8397, 286.8531) (-276.2682, 286.2793) (-276.5882, 285.6026) (-276.8025, 284.8146) (-276.9294, 283.9115) (-276.9938, 282.8973) (-277.0205, 281.7862) (-277.0261, 280.6059) (-277.0209, 279.3903) (-277.0101, 278.173) (-276.9953, 276.9802) (-276.9764, 275.8237) (-276.9527, 274.6943) (-276.9233, 273.5703) (-276.8876, 272.4251) (-276.8459, 271.2354) (-276.7998, 269.9896) (-276.752, 268.6934) (-276.7062, 267.3637) (-276.6661, 266.023) (-276.6346, 264.6938) (-276.6131, 263.3929) (-276.6009, 262.1257) (-276.5953, 260.8864) (-276.5928, 259.6636) (-276.5895, 258.4428) (-276.5818, 257.2108) (-276.5678, 255.9598) (-276.5467, 254.6881) (-276.5191, 253.3978) (-276.4861, 252.0927) (-276.4487, 250.7759) (-276.408, 249.448) (-276.3642, 248.1051) (-276.3174, 246.7412) (-276.2672, 245.3503) (-276.2136, 243.9288) (-276.1564, 242.4774) (-276.0965, 241.0039) (-276.0348, 239.5236) (-275.9729, 238.0552) (-275.9117, 236.6174) (-275.8517, 235.2254) (-275.7925, 233.8875) (-275.7322, 232.6009) (-275.6674, 231.3506) (-275.5943, 230.115) (-275.5092, 228.8705) (-275.4097, 227.5962) (-275.2951, 226.2788) (-275.1678, 224.9172) (-275.0317, 223.5195) (-274.892, 222.0997) (-274.7538, 220.674) (-274.6217, 219.258) (-274.4985, 217.863) (-274.3845, 216.4933) (-274.2787, 215.1483) (-274.1786, 213.8238) (-274.0812, 212.5135) (-273.9836, 211.2107) (-273.8835, 209.9103) (-273.7793, 208.6086) (-273.6701, 207.3036) (-273.5784, 206.2562) (-273.5071, 205.4686) (-273.4585, 204.9425) (-273.4339, 204.6793) knots 0 0 0 0 0 0 0.01428571 0.02857143 0.04285714 0.05714286 0.07142857 0.08571429 0.1 0.11428571 0.12857143 0.14285714 0.15714286 0.17142857 0.18571429 0.2 0.21428571 0.22857143 0.24285714 0.25714286 0.27142857 0.28571429 0.3 0.31428571 0.32857143 0.34285714 0.35714286 0.37142857 0.38571429 0.4 0.41428571 0.42857143 0.44285714 0.45714286 0.47142857 0.48571429 0.5 0.51428571 0.52857143 0.54285714 0.55714286 0.57142857 0.58571429 0.6 0.61428571 0.62857143 0.64285714 0.65714286 0.67142857 0.68571429 0.7 0.71428571 0.72857143 0.74285714 0.75714286 0.77142857 0.78571429 0.8 0.81428571 0.82857143 0.84285714 0.85714286 0.87142857 0.88571429 0.9 0.91428571 0.92857143 0.94285714 0.95714286 0.97142857 0.98571429 1 1 1 1 1 1
  spline S14 degree 5 poles (-268.4687, 204.5782) (-268.435, 204.571) (-268.3676, 204.5553) (-268.2667, 204.5282) (-268.1326, 204.4852) (-267.9668, 204.4186) (-267.8066, 204.3358) (-267.6596, 204.23) (-267.5337, 204.0936) (-267.4347, 203.9206) (-267.3631, 203.7088) (-267.3162, 203.4582) (-267.2893, 203.1698) (-267.2776, 202.8436) (-267.2774, 202.4783) (-267.2853, 202.0724) (-267.2986, 201.6247) (-267.3147, 201.136) (-267.3316, 200.6089) (-267.3469, 200.0498) (-267.3587, 199.4678) (-267.3657, 198.8736) (-267.3672, 198.2788) (-267.3635, 197.6947) (-267.3563, 197.1312) (-267.349, 196.5959) (-267.3466, 196.0933) (-267.3563, 195.6233) (-267.3864, 195.1828) (-267.4453, 194.7667) (-267.5401, 194.3698) (-267.6758, 193.9877) (-267.854, 193.618) (-268.072, 193.2622) (-268.3234, 192.925) (-268.6002, 192.6125) (-268.894, 192.3318) (-269.1976, 192.0896) (-269.5068, 191.8912) (-269.8213, 191.7393) (-270.1431, 191.6351) (-270.4752, 191.5785) (-270.8197, 191.5686) (-271.1765, 191.6049) (-271.5418, 191.6868) (-271.9096, 191.8139) (-272.2719, 191.9846) (-272.6205, 192.1962) (-272.9468, 192.4439) (-273.2439, 192.7206) (-273.506, 193.0173) (-273.7289, 193.3261) (-273.9106, 193.641) (-274.0507, 193.9597) (-274.1514, 194.2862) (-274.2171, 194.6301) (-274.2535, 195.0041) (-274.2673, 195.4208) (-274.2654, 195.8904) (-274.2543, 196.4177) (-274.2396, 196.9994) (-274.2255, 197.6254) (-274.2156, 198.2809) (-274.2125, 198.9483) (-274.2178, 199.609) (-274.2327, 200.2455) (-274.2576, 200.8435) (-274.2924, 201.393) (-274.3364, 201.8915) (-274.3885, 202.3431) (-274.4464, 202.7549) (-274.5063, 203.1337) (-274.5622, 203.4831) (-274.6059, 203.8003) (-274.6258, 204.0714) (-274.6092, 204.2763) (-274.5461, 204.401) (-274.4337, 204.4496) (-274.2799, 204.4539) (-274.0965, 204.4547) (-273.8926, 204.4827) (-273.7165, 204.5382) (-273.5778, 204.6006) (-273.4824, 204.6515) (-273.4339, 204.6793) knots 0 0 0 0 0 0 0.0125 0.025 0.0375 0.05 0.0625 0.075 0.0875 0.1 0.1125 0.125 0.1375 0.15 0.1625 0.175 0.1875 0.2 0.2125 0.225 0.2375 0.25 0.2625 0.275 0.2875 0.3 0.3125 0.325 0.3375 0.35 0.3625 0.375 0.3875 0.4 0.4125 0.425 0.4375 0.45 0.4625 0.475 0.4875 0.5 0.5125 0.525 0.5375 0.55 0.5625 0.575 0.5875 0.6 0.6125 0.625 0.6375 0.65 0.6625 0.675 0.6875 0.7 0.7125 0.725 0.7375 0.75 0.7625 0.775 0.7875 0.8 0.8125 0.825 0.8375 0.85 0.8625 0.875 0.8875 0.9 0.9125 0.925 0.9375 0.95 0.9625 0.975 0.9875 1 1 1 1 1 1
  spline S15 degree 5 poles (-215.0905, 203.3708) (-215.1465, 203.3929) (-215.2541, 203.4268) (-215.4024, 203.4475) (-215.5735, 203.4144) (-215.7432, 203.2715) (-215.8689, 203.0277) (-215.952, 202.6852) (-215.9948, 202.2483) (-216.0007, 201.7229) (-215.9747, 201.117) (-215.9235, 200.4405) (-215.8541, 199.7052) (-215.7737, 198.924) (-215.6881, 198.1112) (-215.6013, 197.2814) (-215.5139, 196.45) (-215.423, 195.6322) (-215.3209, 194.8435) (-215.1977, 194.0983) (-215.0418, 193.4102) (-214.8414, 192.7912) (-214.5856, 192.2513) (-214.2657, 191.7977) (-213.8767, 191.4346) (-213.4159, 191.1638) (-212.9892, 191.0213) (-212.6366, 190.9559) (-212.387, 190.9308) (-212.2586, 190.9228) knots 0 0 0 0 0 0 0.04 0.08 0.12 0.16 0.2 0.24 0.28 0.32 0.36 0.4 0.44 0.48 0.52 0.56 0.6 0.64 0.68 0.72 0.76 0.8 0.84 0.88 0.92 0.96 1 1 1 1 1 1
  spline S16 degree 5 poles (-210.3613, 204.3247) (-210.3119, 204.3026) (-210.2157, 204.255) (-210.0795, 204.1737) (-209.9138, 204.0454) (-209.733, 203.8512) (-209.5778, 203.621) (-209.4459, 203.3507) (-209.3343, 203.0346) (-209.2389, 202.6678) (-209.1549, 202.2476) (-209.0768, 201.7759) (-208.9993, 201.2587) (-208.9171, 200.7049) (-208.826, 200.1247) (-208.7229, 199.5283) (-208.6066, 198.9245) (-208.4784, 198.3192) (-208.3417, 197.716) (-208.2024, 197.1168) (-208.0684, 196.5226) (-207.9497, 195.9346) (-207.8583, 195.3546) (-207.8083, 194.7863) (-207.8147, 194.2351) (-207.8915, 193.7074) (-208.0488, 193.2105) (-208.291, 192.7513) (-208.6145, 192.3359) (-209.0048, 191.9691) (-209.4397, 191.6543) (-209.8942, 191.3933) (-210.3445, 191.1868) (-210.7726, 191.034) (-211.1712, 190.9331) (-211.545, 190.8811) (-211.8321, 190.8762) (-212.0455, 190.892) (-212.1876, 190.9111) (-212.2586, 190.9228) knots 0 0 0 0 0 0 0.028571 0.057143 0.085714 0.114286 0.142857 0.171429 0.2 0.228571 0.257143 0.285714 0.314286 0.342857 0.371429 0.4 0.428571 0.457143 0.485714 0.514286 0.542857 0.571429 0.6 0.628571 0.657143 0.685714 0.714286 0.742857 0.771429 0.8 0.828571 0.857143 0.885714 0.914286 0.942857 0.971429 1 1 1 1 1 1
  line L0 (-210.9023, 190.6998) -> (-213.6149, 191.1458)
  spline S17 degree 5 poles (-215.0905, 203.3708) (-215.0967, 203.4305) (-215.1086, 203.544) (-215.125, 203.697) (-215.1481, 203.9278) (-215.1925, 204.4704) (-215.257, 205.3143) (-215.34, 206.4055) (-215.436, 207.6291) (-215.538, 208.8568) (-215.6398, 209.993) (-215.7384, 211.017) (-215.8332, 211.9579) (-215.9251, 212.8749) (-216.0158, 213.8351) (-216.1073, 214.8932) (-216.2009, 216.0674) (-216.2971, 217.3438) (-216.3961, 218.6877) (-216.4974, 220.0525) (-216.6005, 221.3899) (-216.7042, 222.6587) (-216.8074, 223.836) (-216.9089, 224.9233) (-217.0076, 225.9378) (-217.1022, 226.9074) (-217.192, 227.863) (-217.2764, 228.833) (-217.3552, 229.8354) (-217.4287, 230.8787) (-217.4971, 231.964) (-217.5609, 233.0873) (-217.6203, 234.2416) (-217.6754, 235.4192) (-217.7257, 236.6134) (-217.7708, 237.8182) (-217.8102, 239.028) (-217.844, 240.2377) (-217.8725, 241.442) (-217.8968, 242.6358) (-217.919, 243.8135) (-217.9418, 244.9702) (-217.9676, 246.1022) (-217.9985, 247.208) (-218.0358, 248.2888) (-218.0792, 249.3497) (-218.1266, 250.4005) (-218.1747, 251.4531) (-218.22, 252.521) (-218.2589, 253.6165) (-218.2889, 254.7496) (-218.309, 255.9257) (-218.3203, 257.1454) (-218.3246, 258.4049) (-218.3247, 259.6967) (-218.3231, 261.0103) (-218.3221, 262.3327) (-218.3225, 263.6491) (-218.324, 264.9434) (-218.3248, 266.2004) (-218.3233, 267.4084) (-218.3179, 268.5612) (-218.3084, 269.6608) (-218.2963, 270.7193) (-218.286, 271.7623) (-218.2834, 272.8238) (-218.295, 273.9375) (-218.3257, 275.1286) (-218.378, 276.4052) (-218.4499, 277.7516) (-218.5336, 279.1166) (-218.6164, 280.4269) (-218.6832, 281.6055) (-218.7176, 282.5894) (-218.7046, 283.3472) (-218.6318, 283.8963) (-218.492, 284.3236) (-218.2828, 284.7402) (-218.0071, 285.2254) (-217.6728, 285.78) (-217.2893, 286.3617) (-216.8655, 286.9106) (-216.406, 287.3843) (-215.9112, 287.7606) (-215.38, 288.029) (-214.8106, 288.1858) (-214.3242, 288.2204) (-213.9419, 288.1948) (-213.6792, 288.1549) (-213.5459, 288.1293) knots 0 0 0 0 0 0 0.01176471 0.02352941 0.03529412 0.04705882 0.05882353 0.07058824 0.08235294 0.09411765 0.10588235 0.11764706 0.12941176 0.14117647 0.15294118 0.16470588 0.17647059 0.18823529 0.2 0.21176471 0.22352941 0.23529412 0.24705882 0.25882353 0.27058824 0.28235294 0.29411765 0.30588235 0.31764706 0.32941176 0.34117647 0.35294118 0.36470588 0.37647059 0.38823529 0.4 0.41176471 0.42352941 0.43529412 0.44705882 0.45882353 0.47058824 0.48235294 0.49411765 0.50588235 0.51764706 0.52941176 0.54117647 0.55294118 0.56470588 0.57647059 0.58823529 0.6 0.61176471 0.62352941 0.63529412 0.64705882 0.65882353 0.67058824 0.68235294 0.69411765 0.70588235 0.71764706 0.72941176 0.74117647 0.75294118 0.76470588 0.77647059 0.78823529 0.8 0.81176471 0.82352941 0.83529412 0.84705882 0.85882353 0.87058824 0.88235294 0.89411765 0.90588235 0.91764706 0.92941176 0.94117647 0.95294118 0.96470588 0.97647059 0.98823529 1 1 1 1 1 1
  line L1 (-214.2131, 194.906) -> (-215.9679, 211.8357)
  line L2 (-272.7009, 290.8399) -> (-212.8441, 290.422)
  line L3 (-272.7009, 290.8399) -> (-272.7173, 288.4864)
  line L4 (-254.3875, 290.7121) -> (-254.3567, 288.4328)
  line L5 (-232.7833, 288.3613) -> (-232.7679, 290.5611)
  point P0 (-212.3453, 288.0175)
  point P1 (-211.2196, 287.5177)
  point P2 (-210.2186, 286.7728)
  point P3 (-209.4421, 285.8841)
  point P4 (-208.9363, 284.6731)
  point P5 (-208.6797, 282.983)
  point P6 (-208.6225, 281.5739)
  point P7 (-208.646, 279.8075)
  point P8 (-208.6583, 278.8029)
  point P9 (-208.6698, 277.3427)
  point P10 (-208.7003, 274.1033)
  point P11 (-208.7137, 272.9195)
  point P12 (-208.719, 271.4346)
  point P13 (-208.7101, 270.4996)
  point P14 (-208.6018, 268.1386)
  point P15 (-208.4813, 265.8135)
  point P16 (-208.5032, 262.6805)
  point P17 (-208.5168, 259.1031)
  point P18 (-208.4639, 256.3956)
  point P19 (-208.3864, 252.8062)
  point P20 (-208.3653, 247.0227)
  point P21 (-208.2825, 244.192)
  point P22 (-208.2575, 241.7145)
  point P23 (-208.4397, 236.3586)
  point P24 (-208.7016, 232.1807)
  point P25 (-209.0136, 228.0004)
  point P26 (-209.0415, 225.241)
  point P27 (-209.2161, 222.0986)
  point P28 (-209.5958, 217.3629)
  point P29 (-210.068, 212.2684)
  point P30 (-210.2529, 207.8525)
  point P31 (-210.3881, 205.9735)
  point P32 (-209.67, 203.7483)
  point P33 (-209.2025, 202.4734)
  point P34 (-208.6977, 199.4079)
  point P35 (-207.9024, 195.6067)
  point P36 (-208.3694, 192.6755)
  point P37 (-210.6141, 191.0963)
  point P38 (-215.1484, 203.9503)
  point P39 (-215.5296, 208.7374)
  point P40 (-216.0346, 214.0676)
  point P41 (-216.6786, 222.3332)
  point P42 (-217.2124, 228.1101)
  point P43 (-217.6081, 234.0233)
  point P44 (-217.872, 241.4633)
  point P45 (-218.0353, 248.2284)
  point P46 (-218.274, 254.2374)
  point P47 (-218.3224, 262.3776)
  point P48 (-218.3044, 269.9911)
  point P49 (-218.3977, 276.7283)
  point P50 (-218.6846, 283.365)
  point P51 (-218.2893, 284.7131)
  point P52 (-217.1574, 286.5191)
  point P53 (-215.5266, 287.9357)
  point P54 (-232.1236, 288.3567)
  point P55 (-230.5337, 287.627)
  point P56 (-229.1061, 286.2323)
  point P57 (-228.3804, 284.7374)
  point P58 (-228.2872, 284.0234)
  point P59 (-228.3045, 281.5556)
  point P60 (-228.3918, 277.3338)
  point P61 (-228.382, 273.2077)
  point P62 (-228.2962, 268.9269)
  point P63 (-228.2266, 265.0896)
  point P64 (-228.1623, 260.5004)
  point P65 (-228.1117, 256.7018)
  point P66 (-228.0734, 251.1295)
  point P67 (-228.0652, 246.7913)
  point P68 (-228.0648, 241.3157)
  point P69 (-228.0207, 236.5916)
  point P70 (-228.0637, 233.1986)
  point P71 (-228.2317, 228.4568)
  point P72 (-228.3513, 225.1414)
  point P73 (-228.7104, 220.6515)
  point P74 (-228.9519, 216.4308)
  point P75 (-229.3288, 212.1532)
  point P76 (-229.3877, 209.2422)
  point P77 (-229.4221, 207.0831)
  point P78 (-229.1619, 204.0542)
  point P79 (-228.6861, 203.822)
  point P80 (-228.3947, 202.7676)
  point P81 (-228.4164, 199.6558)
  point P82 (-228.434, 197.145)
  point P83 (-228.4537, 194.3204)
  point P84 (-228.8414, 192.6682)
  point P85 (-229.7421, 191.6187)
  point P86 (-230.3627, 191.3663)
  point P87 (-231.8183, 191.3194)
  point P88 (-232.8023, 191.369)
  point P89 (-234.1098, 192.0915)
  point P90 (-235.0837, 193.5963)
  point P91 (-235.4061, 196.4518)
  point P92 (-235.3921, 200.5034)
  point P93 (-235.7412, 203.6302)
  point P94 (-235.5822, 203.9287)
  point P95 (-235.0817, 204.0956)
  point P96 (-234.9012, 207.7712)
  point P97 (-235.1672, 211.844)
  point P98 (-235.5979, 217.1478)
  point P99 (-235.9647, 221.6889)
  point P100 (-236.3819, 226.4383)
  point P101 (-236.7989, 231.2223)
  point P102 (-237.123, 236.9065)
  point P103 (-237.4466, 242.66)
  point P104 (-237.6439, 249.1401)
  point P105 (-237.6651, 255.283)
  point P106 (-237.8225, 260.0288)
  point P107 (-237.9996, 264.6795)
  point P108 (-238.0673, 268.6435)
  point P109 (-238.1553, 274.3225)
  point P110 (-238.2843, 279.857)
  point P111 (-238.2545, 284.1328)
  point P112 (-237.5921, 285.9308)
  point P113 (-236.0092, 287.4918)
  point P114 (-235.6092, 287.7406)
  point P115 (-250.0308, 189.9043)
  point P116 (-249.4011, 191.9358)
  point P117 (-249.2314, 195.8882)
  point P118 (-249.1126, 199.3437)
  point P119 (-248.8954, 203.3338)
  point P120 (-249.0281, 204.6698)
  point P121 (-251.6557, 189.7569)
  point P122 (-252.3238, 190.4005)
  point P123 (-252.8178, 191.8848)
  point P124 (-253.0648, 195.2987)
  point P125 (-253.3132, 199.0861)
  point P126 (-253.6633, 202.8188)
  point P127 (-253.9409, 203.6204)
  point P128 (-254.1535, 204.1883)
  point P129 (-253.9995, 204.7702)
  point P130 (-253.6653, 204.9178)
  point P131 (-253.2846, 288.3351)
  point P132 (-252.4853, 288.0381)
  point P133 (-251.0951, 287.2901)
  point P134 (-250.1386, 286.2682)
  point P135 (-249.474, 285.3516)
  point P136 (-249.2237, 284.2314)
  point P137 (-249.171, 281.428)
  point P138 (-249.1054, 277.2635)
  point P139 (-248.9463, 272.9469)
  point P140 (-248.8295, 267.9841)
  point P141 (-248.7324, 263.4484)
  point P142 (-248.6619, 260.2896)
  point P143 (-248.5372, 257.0674)
  point P144 (-248.4257, 255.6697)
  point P145 (-248.382, 253.7982)
  point P146 (-248.4068, 250.6518)
  point P147 (-248.284, 246.6207)
  point P148 (-248.17, 241.3218)
  point P149 (-248.1004, 236.1591)
  point P150 (-248.1585, 232.1595)
  point P151 (-248.3727, 227.4214)
  point P152 (-248.7096, 222.4125)
  point P153 (-249.0547, 217.2828)
  point P154 (-249.2756, 212.6806)
  point P155 (-249.5814, 207.7922)
  point P156 (-255.9885, 288.0476)
  point P157 (-257.6668, 286.449)
  point P158 (-258.7382, 284.9598)
  point P159 (-259.0367, 282.8969)
  point P160 (-258.8863, 280.0162)
  point P161 (-258.6863, 276.1122)
  point P162 (-258.5268, 271.8105)
  point P163 (-258.3397, 266.0499)
  point P164 (-258.0951, 260.3837)
  point P165 (-257.8354, 254.1679)
  point P166 (-257.5689, 248.9183)
  point P167 (-257.4145, 244.1658)
  point P168 (-257.2456, 239.0495)
  point P169 (-256.9512, 234.8189)
  point P170 (-256.484, 230.9111)
  point P171 (-255.8378, 225.7914)
  point P172 (-255.2255, 220.6891)
  point P173 (-254.414, 214.801)
  point P174 (-253.6659, 209.6124)
  point P175 (-271.141, 288.3728)
  point P176 (-269.4841, 287.5924)
  point P177 (-268.3495, 286.4209)
  point P178 (-267.5736, 284.4519)
  point P179 (-267.28, 281.8733)
  point P180 (-267.2584, 279.016)
  point P181 (-267.2601, 275.7953)
  point P182 (-267.2004, 272.4391)
  point P183 (-267.1309, 268.9998)
  point P184 (-267.0725, 265.4566)
  point P185 (-267.001, 262.3081)
  point P186 (-266.9921, 259.1185)
  point P187 (-267.0462, 255.8254)
  point P188 (-266.9681, 252.1366)
  point P189 (-266.9392, 248.8326)
  point P190 (-266.873, 244.9257)
  point P191 (-266.9182, 241.4248)
  point P192 (-266.9538, 239.3183)
  point P193 (-267.0865, 235.2518)
  point P194 (-267.2839, 230.8728)
  point P195 (-267.3937, 227.0982)
  point P196 (-267.4708, 222.03)
  point P197 (-267.6967, 216.5666)
  point P198 (-268.0243, 211.4585)
  point P199 (-268.3073, 206.7881)
  point P200 (-274.8033, 287.6649)